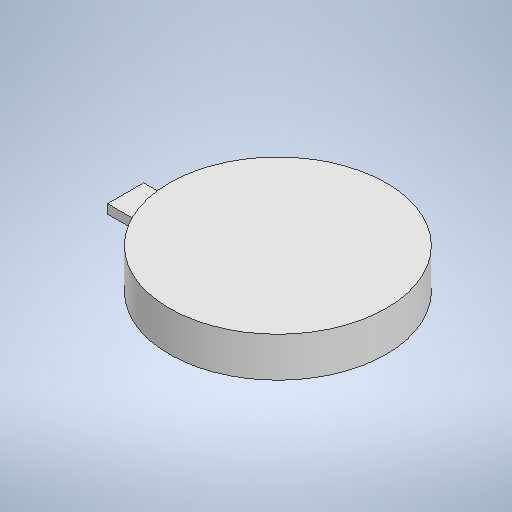
# Autodesk Inventor part: motor
Saved by Autodesk Inventor 2025.2 (Build 292293000, 293)
## iProperties
Created: 2025-08-19
Part Number: motor
Material: 一般
Document SubType Name: Modeling
Designer: naka6
Density: 1 g/cm^3
Appearance: 既定
Author: naka6
Autodesk Inventor part; units mm, degrees
ref_plane "YZ Plane" through (0, 0, 0) normal (1, 0, 0) x (0, 1, 0)
ref_plane "XZ Plane" through (0, 0, 0) normal (0, 1, 0) x (-1, 0, 0)
ref_plane "XY Plane" through (0, 0, 0) normal (0, 0, 1) x (1, 0, 0)
sketch "スケッチ1" plane through (0, 0, 0) normal (0, 1, 0) x (-1, 0, 0)
  circle A0 centre (0, 0) radius 6
  dimension "d0" = 12
  constraints: 1 centre point, 1 coincident
  measures "d0" diameter of A0
extrude "押し出し1" add sketch "スケッチ1" along normal blind 2.2
sketch "スケッチ2" plane through (0, 0, 0) normal (0, -1, 0) x (1, 0, 0)
  circle A0 centre (0, 0) radius 6 projected
  line L0 (-5.9161, 1) -> (-8.4161, 1)
  line L1 (-8.4161, 1) -> (-8.4161, -1)
  line L2 (-8.4161, -1) -> (-5.9161, -1)
  line L3 (-5.9161, -1) -> (-5.9161, 1)
  circle A1 centre (0, 0) radius 6 projected
  dimension "d3" = 2
  dimension "d4" = 2.5
  constraints: 8 end point, 2 parallel, 2 point on circle, 1 horizontal, 1 perpendicular
  measures "d3" distance of L0.end L1.end
  measures "d4" distance of L1.end L2.end
extrude "押し出し2" add sketch "スケッチ2" against normal blind 0.5 contours L3 A0 | A0 L2 L1 L0 picked at (-5.941, 0.1116)
